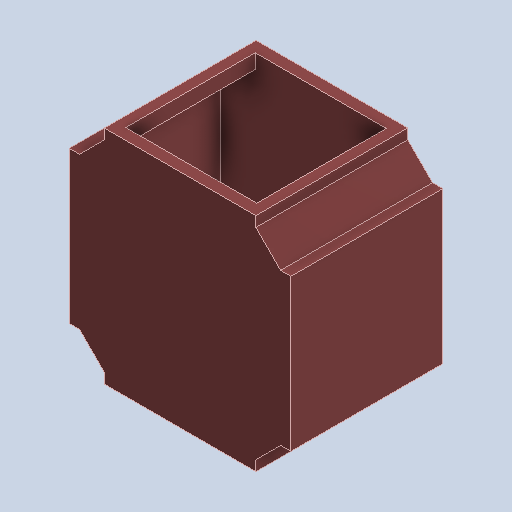
# Autodesk Inventor part: Tunnel Horizontal
Saved by Autodesk Inventor 2023.1 (Build 271208000, 208)
## iProperties
Created: 2022-08-10
Part Number: Tunnel Horizontal
Material: Generic
Document SubType Name: Modeling
Designer: xSibe
Density: 1 g/cm^3
Appearance: Plastic Brown
Author: xSibe
Autodesk Inventor part; units mm, degrees
ref_plane "YZ Plane" through (0, 0, 0) normal (1, 0, 0) x (0, 1, 0)
ref_plane "XZ Plane" through (0, 0, 0) normal (0, 1, 0) x (-1, 0, 0)
ref_plane "XY Plane" through (0, 0, 0) normal (0, 0, 1) x (1, 0, 0)
sketch "Sketch1" plane through (0, 0, 0) normal (0, 0, 1) x (1, 0, 0)
  circle A0 centre (-10, 20.9) radius 1.875 projected
  circle A1 centre (-10, -20.9) radius 1.875 projected
  circle A2 centre (10, 20.9) radius 1.875 projected
  circle A3 centre (10, -20.9) radius 1.875 projected
  circle A4 centre (20.8, -14.4) radius 2.075 projected
  circle A5 centre (20.8, 14.4) radius 2.075 projected
  circle A6 centre (-20.8, 14.4) radius 2.075 projected
  circle A7 centre (-20.8, -14.4) radius 2.075 projected
  line L0 (16.9, -16.9) -> (-16.9, -16.9) projected
  line L1 (-16.9, -16.9) -> (-16.9, 16.9) projected
  line L2 (-16.9, 16.9) -> (16.9, 16.9) projected
  line L3 (16.9, 16.9) -> (16.9, -16.9) projected
  line L4 (-17.05, 24.9) -> (-17.05, 22.55) projected
  line L5 (-17.05, 22.55) -> (-22.55, 17.05) projected
  line L6 (-22.55, 17.05) -> (-24.9, 17.05) projected
  line L7 (-24.9, 17.05) -> (-24.9, -17.05) projected
  line L8 (-24.9, -17.05) -> (-22.55, -17.05) projected
  line L9 (-22.55, -17.05) -> (-17.05, -22.55) projected
  line L10 (-17.05, -22.55) -> (-17.05, -24.9) projected
  line L11 (-17.05, -24.9) -> (17.05, -24.9) projected
  line L12 (17.05, -24.9) -> (17.05, -22.55) projected
  line L13 (17.05, -22.55) -> (22.55, -17.05) projected
  line L14 (22.55, -17.05) -> (24.9, -17.05) projected
  line L15 (24.9, -17.05) -> (24.9, 17.05) projected
  line L16 (24.9, 17.05) -> (22.55, 17.05) projected
  line L17 (22.55, 17.05) -> (17.05, 22.55) projected
  line L18 (17.05, 22.55) -> (17.05, 24.9) projected
  line L19 (17.05, 24.9) -> (-17.05, 24.9) projected
  line L20 (24.825, 16.975) -> (24.825, -16.975)
  line L21 (24.825, -16.975) -> (22.5189, -16.975)
  line L22 (22.5189, -16.975) -> (16.975, -22.5189)
  line L23 (16.975, -22.5189) -> (16.975, -24.825)
  line L24 (16.975, -24.825) -> (-16.975, -24.825)
  line L25 (-16.975, -24.825) -> (-16.975, -22.5189)
  line L26 (-16.975, -22.5189) -> (-22.5189, -16.975)
  line L27 (-22.5189, -16.975) -> (-24.825, -16.975)
  line L28 (-24.825, -16.975) -> (-24.825, 16.975)
  line L29 (-24.825, 16.975) -> (-22.5189, 16.975)
  line L30 (-22.5189, 16.975) -> (-16.975, 22.5189)
  line L31 (-16.975, 22.5189) -> (-16.975, 24.825)
  line L32 (-16.975, 24.825) -> (16.975, 24.825)
  line L33 (16.975, 24.825) -> (16.975, 22.5189)
  line L34 (16.975, 22.5189) -> (22.5189, 16.975)
  line L35 (22.5189, 16.975) -> (24.825, 16.975)
  point P0 (0, 0)
  dimension "d0" = 0.075
  constraints: 32 end point, 15 other
  measures "d0" distance between parallel lines of L15 L20
ref_plane "Work Plane1" through (-24.9, -24.9, 7.7) normal (0, 0, 1) x (1, 0, 0)
extrude "Extrusion1" add sketch "Sketch1" along normal blind 2.5 from surface at 7.7 contours A0 | A1 | A2 | A3 | A4 | A5 | A6 | A7 | L0 L1 L2 L3 | L20 L21 L22 L23 L24 L25 L26 L27 L28 L29 L30 L31 L32 L33 L34 L35
sketch "Sketch2" plane through (0, 0, 0) normal (0, 0, 1) x (1, 0, 0)
  line L0 (22.5189, 16.975) -> (24.825, 16.975) projected
  line L1 (16.975, 22.5189) -> (22.5189, 16.975) projected
  line L2 (16.975, 24.825) -> (16.975, 22.5189) projected
  line L3 (-16.975, 24.825) -> (16.975, 24.825) projected
  line L4 (-16.975, 22.5189) -> (-16.975, 24.825) projected
  line L5 (-22.5189, 16.975) -> (-16.975, 22.5189) projected
  line L6 (-24.825, 16.975) -> (-22.5189, 16.975) projected
  line L7 (-24.825, -16.975) -> (-24.825, 16.975) projected
  line L8 (-22.5189, -16.975) -> (-24.825, -16.975) projected
  line L9 (-16.975, -22.5189) -> (-22.5189, -16.975) projected
  line L10 (-16.975, -24.825) -> (-16.975, -22.5189) projected
  line L11 (16.975, -24.825) -> (-16.975, -24.825) projected
  line L12 (16.975, -22.5189) -> (16.975, -24.825) projected
  line L13 (22.5189, -16.975) -> (16.975, -22.5189) projected
  line L14 (24.825, -16.975) -> (22.5189, -16.975) projected
  line L15 (24.825, 16.975) -> (24.825, -16.975) projected
  line L16 (24.825, -16.975) -> (22.5189, -16.975)
  line L17 (22.5189, -16.975) -> (22.5189, 16.975)
  line L18 (22.5189, 16.975) -> (24.825, 16.975)
  line L19 (24.825, 16.975) -> (24.825, -16.975)
  line L20 (-22.5189, 16.975) -> (-24.825, 16.975)
  line L21 (-24.825, 16.975) -> (-24.825, -16.975)
  line L22 (-24.825, -16.975) -> (-22.5189, -16.975)
  line L23 (-22.5189, -16.975) -> (-22.5189, 16.975)
  line L24 (22.525, -14.675) -> (21.5662, -14.675)
  line L25 (21.5662, -14.675) -> (14.675, -21.5662)
  line L26 (14.675, -21.5662) -> (14.675, -22.525)
  line L27 (14.675, -22.525) -> (-14.675, -22.525)
  line L28 (-14.675, -22.525) -> (-14.675, -21.5662)
  line L29 (-14.675, -21.5662) -> (-21.5662, -14.675)
  line L30 (-21.5662, -14.675) -> (-22.525, -14.675)
  line L31 (-22.525, -14.675) -> (-22.525, 14.675)
  line L32 (-22.525, 14.675) -> (-21.5662, 14.675)
  line L33 (-21.5662, 14.675) -> (-14.675, 21.5662)
  line L34 (-14.675, 21.5662) -> (-14.675, 22.525)
  line L35 (-14.675, 22.525) -> (14.675, 22.525)
  line L36 (14.675, 22.525) -> (14.675, 21.5662)
  line L37 (14.675, 21.5662) -> (21.5662, 14.675)
  line L38 (21.5662, 14.675) -> (22.525, 14.675)
  line L39 (22.525, 14.675) -> (22.525, -14.675)
  line L40 (14.675, 22.525) -> (14.675, 24.825)
  line L41 (-14.675, 22.525) -> (-14.675, 24.825)
  line L42 (-14.675, -22.525) -> (-14.675, -24.825)
  line L43 (14.675, -22.525) -> (14.675, -24.825)
  point P0 (0, 0)
  dimension "d3" = 2.3
  constraints: 56 end point, 6 point on line, 4 parallel, 4 perpendicular, 2 horizontal, 15 other
  measures "d3" distance between parallel lines of L15 L39
extrude "Extrusion2" add sketch "Sketch2" along normal blind 31.5 from surface at 10.2 contours L17 L38 L37 L36 L40 L3 L2 L1 | L0 L15 L14 L17 L24 L39 L38 | L17 L13 L12 L11 L43 L26 L25 L24 | L41 L34 L33 L32 L23 L5 L4 L3 | L42 L11 L10 L9 L23 L30 L29 L28 | L23 L32 L31 L30 L8 L7 L6
extrude "Extrusion3" add sketch "Sketch2" against normal blind 2.5 from surface at 41.7
body "Solid1"
